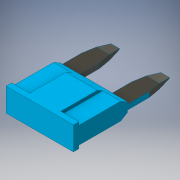
# Autodesk Inventor part: Mini-ATC_FUse
Saved by Autodesk Inventor 2016 (Build 200138000, 138)
## iProperties
Created: 2016-09-30
Part Number: Mini-ATC_FUse
Material: Generic
Document SubType Name: Modeling
Designer: jfixelle
Density: 1 g/cm^3
Appearance: Sky Blue Medium
Author: jfixelle
Autodesk Inventor part; units mm, degrees
ref_plane "YZ Plane" through (0, 0, 0) normal (1, 0, 0) x (0, 1, 0)
ref_plane "XZ Plane" through (0, 0, 0) normal (0, 1, 0) x (-1, 0, 0)
ref_plane "XY Plane" through (0, 0, 0) normal (0, 0, 1) x (1, 0, 0)
sketch "Sketch1" plane through (0, 0, 0) normal (0, 0, 1) x (1, 0, 0)
  line L0 (-5.45, 1.9) -> (5.45, 1.9)
  line L1 (5.45, 1.9) -> (5.45, -1.9)
  line L2 (5.45, -1.9) -> (-5.45, -1.9)
  line L3 (-5.45, -1.9) -> (-5.45, 1.9)
  point P0 (0, 0)
  dimension "d0" = 10.9
  dimension "d1" = 5.45
  dimension "d2" = 3.8
  dimension "d3" = 1.9
  constraints: 8 end point, 2 parallel, 1 horizontal, 1 perpendicular
  measures "d0" distance of L0.start L0.end
  measures "d1" distance from line of point (0, 0) L1
  measures "d2" distance of L0.end L1.end
  measures "d3" distance from line of point (0, 0) L0
extrude "Extrusion1" add sketch "Sketch1" along normal blind 8.8
chamfer "Chamfer1" distance 2 angle 30 1 edges at (0, -1.9, 0) measured on face at (1.8167, -1.9, 2.9333)
chamfer "Chamfer2" distance 2 angle 30 1 edges at (0, 1.9, 0) measured on face at (-1.8167, 1.9, 2.9333)
sketch "Sketch2" plane through (0, 0, 0) normal (0, 0, -1) x (-1, 0, 0)
  line L0 (5.45, -0.4125) -> (2.65, -0.4125)
  line L1 (2.65, -0.4125) -> (2.65, 0.4125)
  line L2 (2.65, 0.4125) -> (5.45, 0.4125)
  line L3 (5.45, 0.4125) -> (5.45, -0.4125)
  line L4 (5.45, -0.7453) -> (5.45, 0.7453) projected
  point P0 (0, 0)
  dimension "d12" = 0
  dimension "d13" = 2.8
  dimension "d14" = 0.825
  dimension "d15" = 0.4125
  constraints: 8 end point, 2 parallel, 1 horizontal, 1 perpendicular
  measures "d12" distance between parallel lines of L4 L3
  measures "d13" distance of L1.end L2.end
  measures "d14" distance of L0.end L1.end
  measures "d15" distance from line of point (0, 0) L0
extrude "Extrusion2" add sketch "Sketch2" along normal blind 7.5
chamfer "Chamfer3" distance 4 angle 10 1 edges at (-5.45, 0, -7.5) measured on face at (-5.45, -0.6333, 4.2667)
chamfer "Chamfer4" distance 4 angle 10 1 edges at (-2.65, 0, -7.5) measured on face at (-2.65, -0.1375, -2.5)
chamfer "Chamfer5" distance 2 angle 10 1 edges at (-4.05, -0.4125, -7.5) measured on face at (-3.8184, -0.4125, -4.8333)
chamfer "Chamfer6" distance 2 angle 10 1 edges at (-4.05, 0.4125, -7.5) measured on face at (-3.8184, 0.4125, -4.8333)
sketch "Sketch3" plane through (-5.45, -1.9, 8.8) normal (0, -1, 0) x (1, 0, 0)
  line L0 (0, -6.8) -> (0, 0) projected
  line L1 (0, -8.8) -> (10.9, -8.8) projected
  line L2 (0, -0.8922) -> (2.9164, -0.8922)
  line L3 (2.9164, -0.8922) -> (2.9164, -8.8)
  line L4 (2.9164, -8.8) -> (0, -8.8)
  line L5 (0, -8.8) -> (0, -0.8922)
  point P0 (5.45, -8.8)
  constraints: 8 end point, 2 parallel, 2 point on line, 1 horizontal, 1 perpendicular
extrude "Extrusion3" cut sketch "Sketch3" against normal blind 0.5
mirror "Mirror1" about plane through (0, 0, 0) normal (0, 1, 0) of "Extrusion3"
mirror "Mirror2" about plane through (0, 0, 0) normal (1, 0, 0) of "Extrusion3", "Mirror1"
mirror "Mirror3" about plane through (0, 0, 0) normal (1, 0, 0) of "Extrusion2"
chamfer "Chamfer7" distance 4 angle 10 1 edges at (2.65, 0, -7.5) measured on face at (2.65, -0.1375, -2.5)
chamfer "Chamfer8" distance 4 angle 10 1 edges at (5.45, 0, -7.5) measured on face at (5.45, 0.4667, 3.3919)
chamfer "Chamfer9" distance 2 angle 10 1 edges at (4.05, 0.4125, -7.5) measured on face at (3.8184, 0.4125, -4.8333)
chamfer "Chamfer10" distance 2 angle 10 1 edges at (4.05, -0.4125, -7.5) measured on face at (3.8184, -0.4125, -4.8333)
body "Solid1"
